massimosquadretta (Autodesk Fusion 360 design; units mm, degrees)
Autodesk Fusion 360 part; units mm, degrees
note: some values were not read from the file. Set by a fixed rule: which sketch regions a step uses.
sketch "support" plane through (0, 0, 0) normal (0, 0, 1) x (1, 0, 0)
  line L0 (20, 10) -> (-20, 10)
  line L1 (-20, 10) -> (-20, -10)
  line L2 (-20, -10) -> (20, -10)
  line L3 (20, -10) -> (20, 10)
  line L4 (20, 10) -> (-20, -10) construction
  line L5 (-20, 10) -> (20, -10) construction
  circle A0 centre (0, 0) radius 6
  line L6 (-20, 0) -> (20, 0)
  circle A1 centre (-13, 0) radius 1.75
  line L7 (0, 10) -> (0, -10)
  circle A2 centre (13, 0) radius 1.75
  circle A3 centre (0, 0) radius 9.2
  dimension "d1" = 40
  dimension "d2" = 20
  dimension "d3" = 12
  dimension "d4" = 3.5
  dimension "d5" = 7
  dimension "d10" = 3.2
  constraint horizontal L0
  constraint perpendicular L0 L1
  constraint parallel L0 L2
  constraint parallel L1 L3
  constraint coincident L4 A0.centre
  constraint coincident L5 A0.centre
  constraint coincident A0.centre A3.centre
  constraint midpoint L1 L6.start
  constraint perpendicular L1 L6
  constraint coincident L6 A1.centre
  constraint midpoint L0 L7.start
  constraint midpoint L2 L7.end
  constraint symmetric A1 L7 A2
  measures "d1" distance of L1.end L2.end
  measures "d2" distance of L0.end L1.end
  measures "d3" diameter of A0
  measures "d4" diameter of A1
  measures "d5" distance of L6.start A1.centre
extrude "Extrude1" add sketch "support" along normal blind 3.2 contours L0 L3 L6 L7 A2 A3 | L0 L1 L6 A1 L7 A3 | L2 L3 L6 L7 A2 A3 | A0 L6 L7 A3 | A0 L6 L7 A3 | L1 L2 L6 A1 L7 A3 | A0 L6 L7 A3 | A0 L6 L7 A3
extrude "Extrude3" add sketch "support" against normal blind 55 contours A0 L6 L7 A3 | A0 L6 L7 A3 | A0 L6 L7 A3 | A0 L6 L7 A3
fillet "Fillet1" radius 2 4 edges at (20, 10, 1.6) (20, -10, 1.6) (-20, 10, 1.6) (-20, -10, 1.6)
named bodies: "Support"
